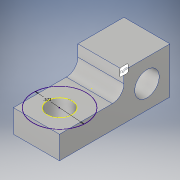
# Autodesk Inventor part: mount
Saved by Autodesk Inventor 2018 (Build 220112000, 112)
## iProperties
Created: 2019-03-04
Part Number: mount
Material: Aluminum 6061
Document SubType Name: Modeling
Designer: freyja
Density: 2.7 g/cm^3
Appearance: Aluminum - Flat
Author: freyja
Autodesk Inventor part; units mm, degrees
ref_plane "YZ Plane" through (0, 0, 0) normal (1, 0, 0) x (0, 1, 0)
ref_plane "XZ Plane" through (0, 0, 0) normal (0, 1, 0) x (-1, 0, 0)
ref_plane "XY Plane" through (0, 0, 0) normal (0, 0, 1) x (1, 0, 0)
sketch "Sketch1" plane through (0, 0, 0) normal (0, 1, 0) x (-1, 0, 0)
  line L0 (-6.35, 15.24) -> (6.35, 15.24)
  line L1 (6.35, 15.24) -> (6.35, -15.24)
  line L2 (6.35, -15.24) -> (-6.35, -15.24)
  line L3 (-6.35, -15.24) -> (-6.35, 15.24)
  line L4 (-6.35, 15.24) -> (6.35, -15.24) construction
  line L5 (6.35, 15.24) -> (-6.35, -15.24) construction
  point P0 (0, 0)
  dimension "d0" = 12.7
  dimension "d1" = 30.48
  constraints: 12 end point, 2 midpoint, 2 parallel, 1 horizontal, 1 perpendicular
  measures "d0" distance of L1.end L2.end
  measures "d1" distance of L0.end L1.end
extrude "Extrusion1" add sketch "Sketch1" along normal blind 12.7
sketch "Sketch2" plane through (0, 12.7, 0) normal (0, 1, 0) x (1, 0, 0)
  line L0 (-6.35, -15.24) -> (6.35, -15.24) projected
  line L1 (0, -15.24) -> (0, -8.89) construction
  point P0 (0, 0)
  dimension "d27" = 6.35
  constraints: 2 end point, 1 coincident, 1 midpoint, 1 vertical
  measures "d27" distance of L1.start L1.end
hole "Hole1" at (0, 12.7, 8.89) direction (0, -1, 0) diameter 6.7564 end through all clearance for "Flat Head Machine Screw (82)" size "1/4" standard "Ansi Unified Screw Threads"
sketch "Sketch3" plane through (-6.35, 0, -15.24) normal (-1, 0, 0) x (0, 0, 1)
  line L0 (0, 0) -> (30.48, 0) projected
  line L1 (0, 0) -> (0, 6.35) construction
  line L2 (0, 0) -> (0, 12.7) projected
  line L3 (0, 6.35) -> (6.35, 6.35) construction
  point P0 (15.24, 0)
  dimension "d12" = 6.35
  dimension "d13" = 6.35
  dimension "d14" = 90
  constraints: 4 end point, 1 coincident, 1 midpoint, 1 perpendicular
  measures "d12" distance of L0.start L1.end
  measures "d13" distance of L1.end L3.end
  measures "d14" angle of L1 L3
hole "Hole2" at (-6.35, 6.35, -8.89) direction (1, 0, 0) diameter 6.7564 end through all clearance for "Flat Head Machine Screw (82)" size "1/4" standard "Ansi Unified Screw Threads"
sketch "Sketch4" plane through (-6.35, 0, -15.24) normal (-1, 0, 0) x (0, 0, 1)
  line L0 (30.48, 0) -> (30.48, 12.7) projected
  line L1 (30.48, 12.7) -> (12.7, 12.7)
  line L2 (12.7, 12.7) -> (12.7, 6.35)
  line L3 (12.7, 6.35) -> (30.48, 6.35)
  line L4 (30.48, 6.35) -> (30.48, 12.7)
  line L5 (0, 0) -> (0, 12.7) projected
  point P0 (15.24, 0)
  dimension "d23" = 6.35
  dimension "d28" = 12.7
  constraints: 8 end point, 2 parallel, 1 horizontal, 1 perpendicular
  measures "d23" distance between parallel lines of L1 L3
  measures "d28" distance between parallel lines of L2 L5
extrude "Extrusion2" cut sketch "Sketch4" against normal up to surface (12.7 mm away)
sketch "Sketch5" plane through (-6.35, 6.35, 15.24) normal (0, 1, 0) x (1, 0, 0)
  circle A0 centre (6.35, 6.35) radius 3.3782 projected
  circle A1 centre (6.35, 6.35) radius 7.2771
  point P0 (6.35, 15.24)
  dimension "d26" = 14.5542
  constraints: 1 centre point, 1 coincident
  measures "d26" diameter of A1
fillet "Fillet1" radius 3.175 1 edges at (0, 6.35, -2.54)
body "Solid1"
